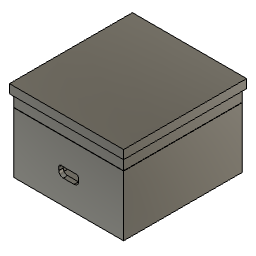
ProjectBox v8 (Autodesk Fusion 360 design; units mm, degrees)
Autodesk Fusion 360 part; units mm, degrees
note: some values were not read from the file. Set by a fixed rule: which sketch regions a step uses.
sketch "Sketch1" plane through (0, 0, 0) normal (0, 0, 1) x (1, 0, 0)
  line L0 (23, 25) -> (-23, 25)
  line L1 (-23, 25) -> (-23, -25)
  line L2 (-23, -25) -> (23, -25)
  line L3 (23, -25) -> (23, 25)
  line L4 (23, 25) -> (-23, -25) construction
  line L5 (-23, 25) -> (23, -25) construction
  line L6 (-25, -27) -> (25, -27)
  line L7 (25, -27) -> (25, 27)
  line L8 (25, 27) -> (-25, 27)
  line L9 (-25, 27) -> (-25, -27)
  dimension "d3" = 46
  dimension "d4" = 50
  dimension "d6" = 2
  constraint horizontal L0
  constraint perpendicular L0 L1
  constraint parallel L0 L2
  constraint parallel L1 L3
  constraint coincident L4 origin
  constraint coincident L5 origin
  measures "d3" distance of L1.end L2.end
  measures "d4" distance of L0.end L1.end
extrude "Extrude1" add sketch "Sketch1" along normal blind 2 contours L0 L1 L2 L3 | L6 L7 L8 L9 makes body 1
extrude "Extrude2" add sketch "Sketch1" along normal blind 33 bodies 1
sketch "Sketch2" plane through (0, 0, 33) normal (0, 0, 1) x (-1, 0, 0)
  line L0 (-23, -25) -> (-23, 25)
  line L1 (-23, 25) -> (23, 25)
  line L2 (23, 25) -> (23, -25)
  line L3 (23, -25) -> (-23, -25)
  line L4 (25, -27) -> (25, 27)
  line L5 (25, 27) -> (-25, 27)
  line L6 (-25, 27) -> (-25, -27)
  line L7 (-25, -27) -> (25, -27)
  line L8 (24, 26) -> (-24, 26)
  line L9 (-24, 26) -> (-24, -26)
  line L10 (-24, -26) -> (24, -26)
  line L11 (24, -26) -> (24, 26)
  line L12 (26, 28) -> (-26, 28)
  line L13 (-26, 28) -> (-26, -28)
  line L14 (-26, -28) -> (26, -28)
  line L15 (26, -28) -> (26, 28)
  line L16 (24.2, -26.2) -> (24.2, 26.2)
  line L17 (24.2, 26.2) -> (-24.2, 26.2)
  line L18 (-24.2, 26.2) -> (-24.2, -26.2)
  line L19 (-24.2, -26.2) -> (24.2, -26.2)
  dimension "d12" = -1
  dimension "d14" = 1
  dimension "d24" = -0.8
extrude "Extrude3" cut sketch "Sketch2" against normal blind 5.5 contours L4 L5 L6 L7 | L16 L17 L18 L19 bodies 1
extrude "Extrude4" add sketch "Sketch2" along normal blind 4 separate body contours L0 L1 L2 L3 | L4 L5 L6 L7 | L8 L9 L10 L11 | L12 L13 L14 L15 | L16 L17 L18 L19 makes body 2
fillet "Fillet1" radius 0.6667 tangency weight 1.2 4 edges at (0, -26, 27.5) (24, 0, 27.5) (0, 26, 27.5) (-24, 0, 27.5) on bodies 1
extrude "Extrude5" add sketch "Sketch2" against normal blind 5.5 contours L4 L5 L6 L7 bodies 2
fillet "Fillet2" radius 0.6667 4 edges at (0, -26.2, 27.5) (24.2, 0, 27.5) (-24.2, 0, 27.5) (0, 26.2, 27.5) on bodies 2
fillet "Fillet3" radius 0.6667 4 edges at (25, 0, 33) (0, -27, 33) (-25, 0, 33) (0, 27, 33) on bodies 2
sketch "Sketch6" plane through (0, 26, 0) normal (0, 1, 0) x (-1, 0, 0)
  line L0 (24, 28.1667) -> (-24, 28.1667)
  line L1 (24, 28.1667) -> (24, 33)
  line L2 (24, 33) -> (-24, 33)
  line L3 (-24, 33) -> (-24, 28.1667)
  line L4 (0, 33) -> (0, 28.1667)
  line L5 (-24, 33) -> (0, 28.1667)
  line L6 (0, 33) -> (-24, 28.1667)
  line L7 (-6.25, 30.0833) -> (-17.75, 30.0833)
  line L8 (-17.75, 30.0833) -> (-17.75, 31.0833)
  line L9 (-17.75, 31.0833) -> (-6.25, 31.0833)
  line L10 (-6.25, 31.0833) -> (-6.25, 30.0833)
  line L11 (-6.25, 30.0833) -> (-17.75, 31.0833) construction
  line L12 (-17.75, 30.0833) -> (-6.25, 31.0833) construction
  line L13 (17.75, 31.0833) -> (6.25, 31.0833)
  line L14 (6.25, 31.0833) -> (6.25, 30.0833)
  line L15 (6.25, 30.0833) -> (17.75, 30.0833)
  line L16 (17.75, 30.0833) -> (17.75, 31.0833)
  point P0 (-12, 30.5833)
  dimension "d35" = 11.5
  dimension "d36" = 1
  constraint midpoint L2 L4.start
  constraint midpoint L0 L4.end
  constraint coincident L2.end L3.start
  constraint coincident L0.end L3.end
  constraint horizontal L7
  constraint perpendicular L7 L8
  constraint parallel L7 L9
  constraint parallel L8 L10
  constraint coincident L11 P0
  constraint coincident L12 P0
  constraint midpoint L6 P0
  constraint symmetric L4 L7.start L14.end
  constraint symmetric L4 L7.end L15.end
  constraint symmetric L4 L8.end L13.start
  constraint symmetric L4 L9.end L13.end
  measures "d35" distance of L8.end L9.end
  measures "d36" distance of L7.end L8.end
sketch "Sketch7" plane through (0, -26, 0) normal (0, -1, 0) x (1, 0, 0)
  line L0 (24, 28.1667) -> (-24, 28.1667)
  line L1 (24, 28.1667) -> (24, 33)
  line L2 (24, 33) -> (-24, 33)
  line L3 (-24, 33) -> (-24, 28.1667)
  line L4 (-17.75, 31.0833) -> (-6.25, 31.0833)
  line L5 (-6.25, 31.0833) -> (-6.25, 30.0833)
  line L6 (-6.25, 30.0833) -> (-17.75, 30.0833)
  line L7 (-17.75, 30.0833) -> (-17.75, 31.0833)
  line L8 (6.25, 31.0833) -> (6.25, 30.0833)
  line L9 (17.75, 31.0833) -> (6.25, 31.0833)
  line L10 (17.75, 30.0833) -> (17.75, 31.0833)
  line L11 (6.25, 30.0833) -> (17.75, 30.0833)
extrude "Extrude8" add sketch "Sketch7" along normal blind 1 draft -50 contours L4 L5 L6 L7 | L8 L9 L10 L11 bodies 1
extrude "Extrude9" add sketch "Sketch6" along normal blind 1 draft -50 contours L5 L6 L7 | L5 L6 L7 L9 L10 | L5 L6 L7 L8 L9 | L5 L6 L9 | L13 L14 L15 L16 bodies 1
sketch "Sketch11" plane through (0, -26.2, 0) normal (0, 1, 0) x (-1, 0, 0)
  line L0 (-24.2, 28.1667) -> (24.2, 28.1667)
  line L1 (24.2, 28.1667) -> (24.2, 33)
  line L2 (24.2, 33) -> (-24.2, 33)
  line L3 (-24.2, 33) -> (-24.2, 28.1667)
  line L4 (-17.75, 31.0833) -> (-6.25, 31.0833)
  line L5 (-6.25, 30.0833) -> (-17.75, 30.0833)
  line L6 (-6.25, 31.0833) -> (-6.25, 30.0833)
  line L7 (-17.75, 30.0833) -> (-17.75, 31.0833)
  line L8 (17.75, 31.0833) -> (6.25, 31.0833)
  line L9 (6.25, 31.0833) -> (6.25, 30.0833)
  line L10 (6.25, 30.0833) -> (17.75, 30.0833)
  line L11 (17.75, 30.0833) -> (17.75, 31.0833)
extrude "Extrude13" cut sketch "Sketch11" against normal blind 1 draft -50 contours L4 L5 L6 L7 | L8 L9 L10 L11 bodies 2
sketch "Sketch12" plane through (0, 26.2, 0) normal (0, -1, 0) x (1, 0, 0)
  line L0 (-24.2, 28.1667) -> (24.2, 28.1667)
  line L1 (24.2, 28.1667) -> (24.2, 33)
  line L2 (24.2, 33) -> (-24.2, 33)
  line L3 (-24.2, 33) -> (-24.2, 28.1667)
  line L4 (-17.75, 31.0833) -> (-6.25, 31.0833)
  line L5 (-17.75, 30.0833) -> (-17.75, 31.0833)
  line L6 (-6.25, 30.0833) -> (-17.75, 30.0833)
  line L7 (-6.25, 31.0833) -> (-6.25, 30.0833)
  line L8 (17.75, 31.0833) -> (6.25, 31.0833)
  line L9 (6.25, 31.0833) -> (6.25, 30.0833)
  line L10 (6.25, 30.0833) -> (17.75, 30.0833)
  line L11 (17.75, 30.0833) -> (17.75, 31.0833)
extrude "Extrude14" cut sketch "Sketch12" against normal blind 1 draft -50 contours L4 L5 L6 L7 | L8 L9 L10 L11 bodies 2
sketch "Sketch16" plane through (0, 0, 2) normal (0, 0, 1) x (-1, 0, 0)
  line L0 (-23, -25) -> (23, -25)
  line L1 (23, -25) -> (23, 25)
  line L2 (23, 25) -> (-23, 25)
  line L3 (-23, 25) -> (-23, -25)
  line L4 (19.575, -22.175) -> (-19.575, -22.175)
  line L5 (-19.575, -22.175) -> (-19.575, 22.175)
  line L6 (-19.575, 22.175) -> (19.575, 22.175)
  line L7 (19.575, 22.175) -> (19.575, -22.175)
  line L8 (19.575, -22.175) -> (-19.575, 22.175) construction
  line L9 (-19.575, -22.175) -> (19.575, 22.175) construction
  circle A0 centre (19.575, -22.175) radius 1
  circle A1 centre (-19.575, -22.175) radius 1
  circle A2 centre (19.575, 22.175) radius 1
  circle A3 centre (-19.575, 22.175) radius 1
  line L10 (-14, -18) -> (14, -18)
  line L11 (14, -18) -> (14, 18)
  line L12 (14, 18) -> (-14, 18)
  line L13 (-14, 18) -> (-14, -18)
  line L14 (-14, -18) -> (14, 18) construction
  line L15 (14, -18) -> (-14, 18) construction
  line L16 (-14, 18) -> (14, 18)
  line L17 (14, 18) -> (14, 25)
  line L18 (14, 25) -> (-14, 25)
  line L19 (-14, 25) -> (-14, 18)
  line L20 (-14, -18) -> (14, -18)
  line L21 (14, -18) -> (14, -25)
  line L22 (14, -25) -> (-14, -25)
  line L23 (-14, -25) -> (-14, -18)
  line L24 (19.575, -22.175) -> (19.575, -10.175)
  line L25 (19.575, 22.175) -> (19.575, 10.175)
  line L26 (14, -10) -> (19.575, -10)
  line L27 (19.575, -10) -> (19.575, 10.175)
  line L28 (19.575, 10.175) -> (14, 10.175)
  line L29 (14, 10.175) -> (14, -10)
  line L30 (-19.575, -22.175) -> (-19.575, -10.175)
  line L31 (-19.575, 22.175) -> (-19.575, 10.175)
  line L32 (-19.575, -10.175) -> (-14, -10.175)
  line L33 (-14, -10.175) -> (-14, 10)
  line L34 (-14, 10) -> (-19.575, 10)
  line L35 (-19.575, 10) -> (-19.575, -10.175)
  dimension "d76" = 39.15
  dimension "d77" = 44.35
  dimension "d78" = 2
  dimension "d79" = 2
  dimension "d80" = 2
  dimension "d81" = 2
  dimension "d102" = 12
  dimension "d103" = 12
  dimension "d104" = 12
  dimension "d105" = 12
  constraint horizontal L4
  constraint perpendicular L4 L5
  constraint parallel L4 L6
  constraint parallel L5 L7
  constraint coincident L8 origin
  constraint coincident L9 origin
  constraint coincident L4.start L7.end
  constraint coincident L4.end L5.start
  constraint coincident L6.end L7.start
  constraint coincident L5.end L6.start
  constraint horizontal L10
  constraint perpendicular L10 L11
  constraint parallel L10 L12
  constraint parallel L11 L13
  constraint coincident L14 origin
  constraint coincident L15 origin
  constraint horizontal L16
  constraint vertical L17
  constraint horizontal L18
  constraint vertical L19
  constraint coincident L2 L17.end
  constraint horizontal L20
  constraint vertical L21
  constraint horizontal L22
  constraint vertical L23
  constraint coincident L0 L21.end
  constraint perpendicular L4 L24
  constraint perpendicular L6 L25
  constraint horizontal L26
  constraint vertical L27
  constraint horizontal L28
  constraint vertical L29
  constraint coincident L11 L26.start
  constraint parallel L5 L30
  constraint perpendicular L6 L31
  constraint horizontal L32
  constraint vertical L33
  constraint horizontal L34
  constraint vertical L35
  constraint coincident L13 L33.end
  measures "d76" distance of L5.end L6.end
  measures "d77" distance of L4.end L5.end
  measures "d78" diameter of A0
  measures "d79" diameter of A1
  measures "d80" diameter of A2
  measures "d81" diameter of A3
  measures "d102" distance of L4.start L24.end
  measures "d103" distance of L6.end L25.end
  measures "d104" distance of L4.end L30.end
  measures "d105" distance of L5.end L31.end
extrude "Extrude17" add sketch "Sketch16" along normal blind 3.5 contours L0 L2 L3 L4 L5 L6 A1 A3 L19 L23 L30 L31 L35 | L0 L4 L21 L22 L23 | L0 L1 L2 L4 L6 L7 A0 A2 L17 L21 L24 L25 L27 | L4 L5 A1 L13 L23 L30 L32 | L2 L6 L17 L18 L19 | L4 L7 A0 L11 L21 L24 L26 | L5 L6 A3 L13 L19 L31 L34 | L6 L7 A2 L11 L17 L25 L28 bodies 1
sketch "Sketch17" plane through (0, -25, 0) normal (0, 1, 0) x (-1, 0, 0)
  line L0 (-23, 5.5) -> (23, 5.5)
  line L1 (23, 5.5) -> (23, 33)
  line L2 (23, 33) -> (-23, 33)
  line L3 (-23, 33) -> (-23, 5.5)
  line L4 (4.5, 15.5) -> (-4.5, 15.5)
  line L5 (-4.5, 14.5) -> (-4.5, 13)
  line L6 (-4.5, -4.5) -> (4.5, -4.5)
  line L7 (4.5, 13) -> (4.5, 14.5)
  line L8 (4.5, 15.5) -> (-4.5, -4.5) construction
  line L9 (-4.5, 15.5) -> (4.5, -4.5) construction
  line L10 (4.5, 6.5) -> (4.5, 15.5)
  line L11 (3.5, 15.5) -> (-3.5, 15.5)
  arc A0 (4.5, 14.5) -> (3.5, 15.5) centre (3.5, 14.5) ccw
  line L12 (0, 5.5) -> (0, 11)
  line L13 (0, 11) -> (-2.5, 11)
  line L14 (0, 11) -> (2.5, 11)
  arc A1 (-4.5, 13) -> (-2.5, 11) centre (-2.5, 13) ccw
  arc A2 (2.5, 11) -> (4.5, 13) centre (2.5, 13) ccw
  arc A3 (-3.5, 15.5) -> (-4.5, 14.5) centre (-3.5, 14.5) ccw
  point P0 (0, 5.5)
  dimension "d84" = 9
  dimension "d85" = 20
  dimension "d88" = 1
  dimension "d106" = 5.5
  dimension "d108" = 2
  dimension "d109" = 1
  constraint horizontal L4
  constraint perpendicular L4 L5
  constraint parallel L4 L6
  constraint parallel L5 L7
  constraint coincident L8 P0
  constraint coincident L9 P0
  constraint midpoint L0 P0
  constraint vertical L10
  constraint horizontal L11
  constraint coincident L4.start L11
  constraint coincident L4.start L7
  constraint tangent L11 A0
  constraint tangent L7 A0
  constraint coincident P0 L12.start
  constraint perpendicular L0 L12
  constraint coincident L6.end L7
  constraint perpendicular L5 L13
  constraint perpendicular L10 L14
  constraint coincident L6.start L5
  constraint tangent L5 A1
  constraint tangent L13 A1
  constraint tangent L14 A2
  constraint tangent L7 A2
  constraint equal A1 A2
  constraint coincident L4.end L5
  constraint tangent L5 A3
  constraint tangent L11 A3
  measures "d84" distance of L6.start L6.end
  measures "d85" distance of L4.end L6.start
  measures "d88" radius of A0
  measures "d106" distance of P0 L12.end
  measures "d108" radius of A1
  measures "d109" radius of A3
extrude "Extrude18" cut sketch "Sketch17" against normal blind 2 contours L4 L5 L7 L10 L11 A0 L13 L14 A1 A2 A3 bodies 1
sketch "Sketch21" plane through (-25, 0, 0) normal (-1, 0, 0) x (0, -1, 0)
  line L0 (27, 27.5) -> (-27, 27.5)
  line L1 (-27, 27.5) -> (-27, 0)
  line L2 (-27, 0) -> (27, 0)
  line L3 (27, 0) -> (27, 27.5)
  line L4 (25, 5.5) -> (-25, 5.5)
  line L5 (0, 27.5) -> (0, 24.5)
  circle A0 centre (0, 18.88) radius 5.62
  dimension "d100" = 3
  dimension "d101" = 11.24
  constraint midpoint L0 L5.start
  constraint perpendicular L0 L5
  constraint coincident L5.end A0
  measures "d100" distance of L5.start L5.end
  measures "d101" diameter of A0
extrude "Extrude20" cut sketch "Sketch21" against normal blind 2 contours A0 bodies 1
sketch "Sketch23" plane through (0, 0, 33) normal (0, 0, 1) x (-1, 0, 0)
  line L0 (-24, -26) -> (24, -26)
  line L1 (24, -26) -> (24, 26)
  line L2 (24, 26) -> (-24, 26)
  line L3 (-24, 26) -> (-24, -26)
  line L4 (-23, -25) -> (-23, 25)
  line L5 (-23, 25) -> (23, 25)
  line L6 (23, 25) -> (23, -25)
  line L7 (23, -25) -> (-23, -25)
  line L8 (-24, 26) -> (24, 26)
  line L9 (24, 26) -> (24, -26)
  line L10 (24, -26) -> (-24, -26)
  line L11 (-24, -26) -> (-24, 26)
  line L12 (0, 26) -> (0, 21.6)
  line L13 (0, -26) -> (0, -21.5)
  circle A0 centre (19.575, -22.175) radius 1
  circle A1 centre (-19.575, -22.175) radius 1
  circle A2 centre (19.575, 22.175) radius 1
  circle A3 centre (-19.575, 22.175) radius 1
  line L14 (19.575, -22.175) -> (-19.575, -22.175)
  line L15 (-19.575, -22.175) -> (-19.575, 22.175)
  line L16 (-19.575, 22.175) -> (19.575, 22.175)
  line L17 (19.575, 22.175) -> (19.575, -22.175)
  circle A4 centre (19.575, 22.175) radius 1.2
  circle A5 centre (19.575, -22.175) radius 1.2
  circle A6 centre (-19.575, -22.175) radius 1.2
  circle A7 centre (-19.575, 22.175) radius 1.2
  circle A8 centre (19.575, -22.175) radius 2.95
  circle A9 centre (-19.575, -22.175) radius 2.95
  circle A10 centre (19.575, 22.175) radius 2.95
  circle A11 centre (-19.575, 22.175) radius 2.95
  line L18 (-21.575, -24.175) -> (-21.575, 24.175)
  line L19 (-21.575, 24.175) -> (21.575, 24.175)
  line L20 (21.575, 24.175) -> (21.575, -24.175)
  line L21 (21.575, -24.175) -> (-21.575, -24.175)
  dimension "d112" = 4.4
  dimension "d134" = 2.4
  dimension "d135" = 2.4
  dimension "d136" = 2.4
  dimension "d137" = 2.4
  dimension "d138" = 5.9
  dimension "d139" = 5.9
  dimension "d140" = 5.9
  dimension "d141" = 5.9
  dimension "d146" = -2
  constraint horizontal L8
  constraint vertical L9
  constraint horizontal L10
  constraint vertical L11
  constraint coincident L0.end L1.start
  constraint coincident L2.end L3.start
  constraint midpoint L8 L12.start
  constraint perpendicular L8 L12
  constraint horizontal L14
  constraint vertical L15
  constraint horizontal L16
  constraint vertical L17
  constraint coincident A3.centre L15.end
  constraint coincident A0.centre L14.start
  constraint coincident A2.centre L16.end
  constraint concentric A1 A6
  constraint concentric A3 A7
  constraint concentric A0 A8
  constraint concentric A1 A9
  constraint concentric A2 A10
  measures "d112" distance of L12.start L12.end
  measures "d134" diameter of A4
  measures "d135" diameter of A5
  measures "d136" diameter of A6
  measures "d137" diameter of A7
  measures "d138" diameter of A8
  measures "d139" diameter of A9
  measures "d140" diameter of A10
  measures "d141" diameter of A11
extrude "Extrude21" [rolled back] taper angle 0
sketch "Sketch24" plane through (0, 0, 37) normal (0, 0, 1) x (-1, 0, 0)
  line L0 (26, -28) -> (26, 28)
  line L1 (26, 28) -> (-26, 28)
  line L2 (-26, 28) -> (-26, -28)
  line L3 (-26, -28) -> (26, -28)
  circle A0 centre (19.575, 22.175) radius 1.2
  circle A1 centre (19.575, -22.175) radius 1.2
  circle A2 centre (-19.575, -22.175) radius 1.2
  circle A3 centre (-19.575, 22.175) radius 1.2
  circle A4 centre (-19.575, 22.175) radius 2.45
  circle A5 centre (19.575, 22.175) radius 2.45
  circle A6 centre (19.575, -22.175) radius 2.45
  circle A7 centre (-19.575, -22.175) radius 2.45
  dimension "d142" = 4.9
  dimension "d143" = 4.9
  dimension "d144" = 4.9
  dimension "d145" = 4.9
  constraint concentric A3 A4
  constraint concentric A0 A5
  constraint concentric A1 A6
  constraint concentric A2 A7
  measures "d142" diameter of A4
  measures "d143" diameter of A5
  measures "d144" diameter of A6
  measures "d145" diameter of A7
extrude "Extrude22" [rolled back] taper angle 0
extrude "Extrude23" [rolled back] taper angle 0
fillet "Fillet4" [rolled back] radius 1
equation "BoxLength = CircuitLength + 2 * Tolerance"
equation "BoxWidth = CircuitWidth + 2 * Tolerance"
equation "d3 = BoxWidth"
equation "d4 = BoxLength"
equation "WallThickness = 2 mm"
equation "d6 = WallThickness"
equation "BoxHeight = 33 mm"
equation "d8 = WallThickness"
equation "d10 = BoxHeight"
equation "d12 = -WallThickness / 2"
equation "d15 = -OverlapDepth"
equation "LidHeight = WallThickness * 2"
equation "d18 = LidHeight"
equation "d21 = Fillet"
equation "d22 = -OverlapDepth"
equation "d24 = -WallThickness / 2 + 0.2 mm"
equation "d26 = Fillet"
equation "d28 = Fillet"
equation "d35 = NubLength"
equation "NubLength = ( BoxWidth / 4 mm ) * 1 mm"
equation "OverlapDepth = BoxHeight / 6"
equation "Fillet = WallThickness / 3"
equation "MicroUSBBaseHeight = 10 mm"
equation "MicroUSBHeight = 6 mm"
equation "MicroUSBWidth = 10 mm"
equation "WireShortDistanceWall = 2 mm"
equation "WireLongDistanceWall = 13 mm"
equation "WireSpacingLength = 15 mm"
equation "WireSpacingWidth = 8 mm"
equation "Tolerance = 0.5 mm"
equation "CircuitLength = 49 mm"
equation "CircuitWidth = 45 mm"
equation "d86 = -WallThickness"
equation "d98 = -WallThickness"
equation "BigScrewSize = 2.4 mm"
equation "d112 = BigScrewSize + 2 mm"
equation "d117 = -( ScrewHeight - LidHeight )"
equation "ScrewHeight = 10.5 mm"
equation "BigScrewHeadSize = BigScrewSize + 2.5 mm"
equation "BigScrewHeadHeight = 3 mm"
equation "d126 = -BigScrewHeadHeight"
equation "d128 = -LidHeight"
equation "d134 = BigScrewSize"
equation "d135 = BigScrewSize"
equation "d136 = BigScrewSize"
equation "d137 = BigScrewSize"
equation "d138 = BigScrewSize + BigScrewBorder"
equation "d139 = BigScrewSize + BigScrewBorder"
equation "d140 = BigScrewSize + BigScrewBorder"
equation "d141 = BigScrewSize + BigScrewBorder"
equation "d142 = BigScrewHeadSize"
equation "d143 = BigScrewHeadSize"
equation "d144 = BigScrewHeadSize"
equation "d145 = BigScrewHeadSize"
equation "BigScrewBorder = 3.5 mm"
named bodies: "Base", "Lid"
